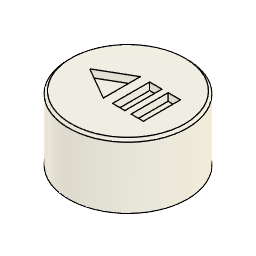
keycap_circle (Autodesk Fusion 360 archive; units mm, degrees)
design "keyCAp"
Autodesk Fusion 360 part; units mm, degrees
sketch "スケッチ1" plane through (0, 0, 0) normal (0, 0, 1) x (1, 0, 0)
  line L0 (-3.5, 3.5) -> (3.5, 3.5)
  line L1 (3.5, 3.5) -> (3.5, -3.5)
  line L2 (3.5, -3.5) -> (-3.5, -3.5)
  line L3 (-3.5, -3.5) -> (-3.5, 3.5)
  line L4 (-3.5, 0) -> (3.5, 0)
  line L5 (-2.5, 2.5) -> (2.5, 2.5)
  line L6 (2.5, 2.5) -> (2.5, -2.5)
  line L7 (2.5, -2.5) -> (-2.5, -2.5)
  line L8 (-2.5, -2.5) -> (-2.5, 2.5)
  line L9 (0, 2.5) -> (0, -2.5)
  line L10 (1.7587, 2.5) -> (0.283, 0.9795)
  line L11 (0.283, 0.9795) -> (1.0007, 0.283)
  line L12 (1.0007, 0.283) -> (2.5, 1.828)
  circle A0 centre (0.9901, 0.9901) radius 0.5
  line L13 (0.9901, 0.9901) -> (2.5, 2.5)
  dimension "d1" = 7
  dimension "d2" = 7
  dimension "d3" = 1
  dimension "d4" = 1
  dimension "d5" = 0.9
  dimension "d6" = 135
  constraint horizontal L0
  constraint vertical L1
  constraint horizontal L2
  constraint vertical L3
  constraint midpoint L3 L4.start
  constraint midpoint L1 L4.end
  constraint midpoint origin L4
  constraint horizontal L5
  constraint vertical L6
  constraint horizontal L7
  constraint vertical L8
  constraint equal L5 L6
  constraint coincident L5 L9.start
  constraint coincident L7 L9.end
  constraint perpendicular L7 L9
  constraint midpoint L5 L9.start
  constraint midpoint L4 L9
  constraint coincident L5 L10.start
  constraint perpendicular L10 L11
  constraint coincident L6 L12.end
  constraint perpendicular L11 L12
  constraint tangent L11 A0
  constraint tangent L12 A0
  constraint tangent L10 A0
  constraint coincident A0.centre L13.start
  measures "d1" distance of L0.start L0.end
  measures "d2" distance of L0.end L1.end
  measures "d3" distance of L0 L5
  measures "d4" distance of L10.end L11.end
  measures "d5" distance of origin L11
  measures "d6" angle of L6 L13
ref_plane "作業平面1" through (0, 0, 3.5) normal (0, 0, 1) x (1, 0, 0)
sketch "スケッチ2" plane through (0, 0, 3.5) normal (0, 0, 1) x (1, 0, 0)
  line L0 (-2.5, 2.5) -> (2.5, 2.5)
  line L1 (2.5, 2.5) -> (2.5, -2.5)
  line L2 (2.5, -2.5) -> (-2.5, -2.5)
  line L3 (-2.5, -2.5) -> (-2.5, 2.5)
  line L4 (-3.5, 3.5) -> (3.5, 3.5)
  line L5 (3.5, 3.5) -> (3.5, -3.5)
  line L6 (3.5, -3.5) -> (-3.5, -3.5)
  line L7 (-3.5, -3.5) -> (-3.5, 3.5)
  line L8 (-2.5, 0) -> (2.5, 0)
  line L9 (0, 3.5) -> (0, -3.5)
  line L10 (2.5, 2.5) -> (0.8132, 0.8132)
  line L11 (2.5, 2.5) -> (4.2, 2.5) construction
  circle A0 centre (0.8132, 0.8132) radius 0.5
  line L12 (1.7929, 2.5) -> (0.4596, 1.1667)
  line L13 (2.5, 1.7929) -> (1.1667, 0.4596)
  line L14 (0, 0) -> (0.4596, 0.4596)
  dimension "d8" = 7
  dimension "d9" = 1
  dimension "d10" = 135
  dimension "d12" = 1
  dimension "d25" = 0.65
  constraint horizontal L0
  constraint vertical L1
  constraint horizontal L2
  constraint vertical L3
  constraint horizontal L4
  constraint vertical L5
  constraint horizontal L6
  constraint vertical L7
  constraint equal L4 L7
  constraint equal L0 L3
  constraint midpoint L3 L8.start
  constraint midpoint L1 L8.end
  constraint midpoint L14.start L8
  constraint midpoint L4 L9.start
  constraint midpoint L6 L9.end
  constraint midpoint L14.start L9
  constraint horizontal L11
  constraint coincident L10.end A0.centre
  constraint coincident L0 L12.start
  constraint coincident A0 L12.end
  constraint tangent A0 L12
  constraint coincident L1 L13.start
  constraint coincident A0 L13.end
  constraint tangent A0 L13
  constraint parallel L10 L13
  constraint parallel L10 L12
  constraint coincident L14.start origin
  constraint coincident A0 L14.end
  constraint collinear L10 L14
  measures "d8" distance of L4.start L6.end
  measures "d9" distance of L0 L4
  measures "d10" angle of L10 L11
  measures "d12" diameter of A0
  measures "d25" distance of L14.start L14.end
loft "ロフト1" add profiles "スケッチ2", "スケッチ1" section 1 contours A0 section 2 contours A0 makes body 1
loft "ロフト2" add profiles "スケッチ1", "スケッチ2" section 1 contours L6 L12 A0 L13 | L5 L10 A0 L13 section 2 contours L0 L10 A0 L12 | L1 L10 A0 L13 separate body makes body 2
combine "結合1" operation add target body 1 tool bodies 2
extrude "押し出し1" add sketch "スケッチ1" along normal blind 3.5 contours L0 L1 L3 L4 L5 L6 L8 | L1 L2 L3 L4 L6 L7 L8 bodies 1
chamfer "面取り1" distance 0.5 angle 45 2 edges at (1.7758, 2.5, 1.75) (2.5, 1.8104, 1.75) on bodies 1
pattern_circular "C パターン2" count 4 over 360 about axis through (0, 0, 1.75) along (0, 0, 1) of bodies 1 makes body 3 at (-1.1335, 1.835, 2.3333) makes body 4 at (-1.835, -1.1335, 2.3333) makes body 5 at (1.1335, -1.835, 2.3333)
combine "結合2" operation add target body 1 tool bodies 3 5 4
sketch "スケッチ3" plane through (0, 0, 3.5) normal (0, 0, 1) x (-1, 0, 0)
  line L0 (3.5, 3.5) -> (-3.5, 3.5)
  line L1 (-3.5, 3.5) -> (-3.5, -3.5)
  line L2 (-3.5, -3.5) -> (3.5, -3.5)
  line L3 (3.5, -3.5) -> (3.5, 3.5)
  line L4 (2.1464, -1.4393) -> (2.5, -1.2929)
  line L5 (2.1464, -1.4393) -> (1.1667, -0.4596)
  arc A0 (1.1667, -0.4596) -> (0.4596, -1.1667) centre (0.8132, -0.8132) ccw
  line L6 (0.4596, -1.1667) -> (1.4393, -2.1464)
  line L7 (1.2929, -2.5) -> (1.4393, -2.1464)
  line L8 (1.2929, -2.5) -> (-1.2929, -2.5)
  line L9 (-1.4393, -2.1464) -> (-1.2929, -2.5)
  line L10 (-1.4393, -2.1464) -> (-0.4596, -1.1667)
  arc A1 (-0.4596, -1.1667) -> (-1.1667, -0.4596) centre (-0.8132, -0.8132) ccw
  line L11 (-1.1667, -0.4596) -> (-2.1464, -1.4393)
  line L12 (-2.5, -1.2929) -> (-2.1464, -1.4393)
  line L13 (-2.5, -1.2929) -> (-2.5, 1.2929)
  line L14 (-2.1464, 1.4393) -> (-2.5, 1.2929)
  line L15 (-2.1464, 1.4393) -> (-1.1667, 0.4596)
  arc A2 (-1.1667, 0.4596) -> (-0.4596, 1.1667) centre (-0.8132, 0.8132) ccw
  line L16 (-0.4596, 1.1667) -> (-1.4393, 2.1464)
  line L17 (-1.2929, 2.5) -> (-1.4393, 2.1464)
  line L18 (-1.2929, 2.5) -> (1.2929, 2.5)
  line L19 (1.4393, 2.1464) -> (1.2929, 2.5)
  line L20 (1.4393, 2.1464) -> (0.4596, 1.1667)
  arc A3 (0.4596, 1.1667) -> (1.1667, 0.4596) centre (0.8132, 0.8132) ccw
  line L21 (1.1667, 0.4596) -> (2.1464, 1.4393)
  line L22 (2.5, 1.2929) -> (2.1464, 1.4393)
  line L23 (2.5, 1.2929) -> (2.5, -1.2929)
extrude "押し出し2" add sketch "スケッチ3" along normal blind 1.5 contours L0 L1 L2 L3 | L4 L5 A0 L6 L7 L8 L9 L10 A1 L11 L12 L13 L14 L15 A2 L16 L17 L18 L19 L20 A3 L21 L22 L23 bodies 1
sketch "スケッチ5" plane through (0, 0, 5) normal (0, 0, 1) x (-1, 0, 0)
  line L0 (3.5, -3.5) -> (3.5, 3.5)
  line L1 (3.5, 3.5) -> (-3.5, 3.5)
  line L2 (-3.5, 3.5) -> (-3.5, -3.5)
  line L3 (-3.5, -3.5) -> (3.5, -3.5)
  circle A0 centre (0, 0) radius 3.81
  dimension "d26" = 7.62
  constraint coincident A0.centre origin
  measures "d26" diameter of A0
extrude "押し出し4" cut sketch "スケッチ5" against normal blind 5 contours L0 L3 A0 | L0 L1 A0 | L2 L3 A0 | L1 L2 A0 bodies 1
extrude "押し出し5" add sketch "スケッチ5" against normal blind 5 contours L0 A0 | L3 A0 | L1 A0 | L2 A0 bodies 1
sketch "スケッチ6" plane through (0, 0, 5) normal (0, 0, 1) x (-1, 0, 0)
  circle A0 centre (0, 0) radius 3.81
  line L0 (0.5, 1.5) -> (0.5, -1.5)
  line L1 (0.5, -1.5) -> (3.0981, 0)
  line L2 (3.0981, 0) -> (0.5, 1.5)
  line L3 (-2.75, 1.5) -> (-1.75, 1.5)
  line L4 (-1.75, 1.5) -> (-1.75, -1.5)
  line L5 (-1.75, -1.5) -> (-2.75, -1.5)
  line L6 (-2.75, -1.5) -> (-2.75, 1.5)
  line L7 (-1.25, -1.5) -> (-1.25, 1.5)
  line L8 (-0.25, -1.5) -> (-1.25, -1.5)
  line L9 (-0.25, 1.5) -> (-0.25, -1.5)
  line L10 (-1.25, 1.5) -> (-0.25, 1.5)
  line L11 (-1.25, 0) -> (-1.75, 0)
  line L12 (-2.75, 0) -> (0, 0)
  point P0 (0.5, 0)
  dimension "d31" = 0.5
  dimension "d32" = 1
  dimension "d33" = 3
  dimension "d34" = 3
  dimension "d36" = 3
  dimension "d41" = 0.25
  dimension "d42" = 0.5
  constraint vertical L0
  constraint horizontal L3
  constraint vertical L4
  constraint horizontal L5
  constraint vertical L6
  constraint midpoint L0 P0
  constraint horizontal L1.end P0
  constraint horizontal A0.centre L1.end
  constraint horizontal L10
  constraint vertical L9
  constraint horizontal L8
  constraint vertical L7
  constraint equal L3 L10
  constraint equal L6 L7
  constraint midpoint L7 L11.start
  constraint midpoint L4 L11.end
  constraint horizontal L11
  constraint midpoint L6 L12.start
  constraint coincident A0.centre L12.end
  constraint horizontal L12
  measures "d31" distance of L4 L7
  measures "d32" distance of L3.start L3.end
  measures "d33" distance of L9.start L8.start
  measures "d34" distance of L0.start L0.end
  measures "d36" distance of L0.start L1.end
  measures "d41" distance of A0.centre L9
  measures "d42" distance of A0.centre L0
extrude "押し出し6" cut sketch "スケッチ6" against normal blind 0.4 contours L0 L1 L2 | L3 L4 L6 L12 | L4 L5 L6 L12 | L7 L8 L9 L12 | L7 L9 L10 L12 bodies 1
move_face "面をオフセット1" offset 1 1 faces at (-3.5707, -1.329, 1.6667) on bodies 1
extrude "押し出し7" add 1 faces at (-2.4201, -1.5395, 5) along direction (0, 0, 1) blind 0.2 on bodies 1 bodies 1
chamfer "面取り2" distance 0.2 angle 45 1 edges at (4.4845, 1.7394, 5.2) on bodies 1
equation "d2 = d1"
